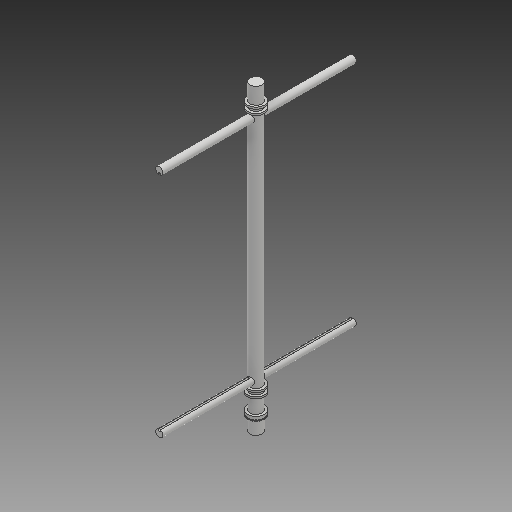
# Autodesk Inventor part: CentralBeam
Saved by Autodesk Inventor 2018 (Build 220112000, 112)
## iProperties
Created: 2016-02-23
Part Number: CentralBeam
Material: Generic
Document SubType Name: Modeling
Designer: Tore Den Store
Density: 1 g/cm^3
Appearance: Default
Author: Tore Den Store
Autodesk Inventor part; units mm, degrees
sketch "Sketch1" plane through (0, 0, 0) normal (0, 0, 1) x (1, 0, 0)
  circle A0 centre (0, 0) radius 50
  dimension "d0" = 100
  constraints: 1 centre point, 1 coincident
  measures "d0" diameter of A0
extrude "Extrusion1" add sketch "Sketch1" along normal blind 3500
ref_plane "Work Plane1" through (0, 0, 1750) normal (0, 0, -1) x (-1, 0, 0)
sketch "Sketch7" plane through (0, 0, 1750) normal (0, 0, -1) x (-1, 0, 0)
  circle A0 centre (0, 0) radius 50
  circle A1 centre (0, 0) radius 70
  constraints: 2 centre point
extrude "Extrusion6" add sketch "Sketch7" along normal blind 25
sketch "Sketch8" plane through (0, 0, 1725) normal (0, 0, -1) x (-1, 0, 0)
  circle A0 centre (0, 0) radius 70
  circle A1 centre (0, 0) radius 50
  line L0 (0, 0) -> (-2.7482, 69.946)
  line L1 (0, 0) -> (2.7482, 69.946)
  line L2 (0, 0) -> (0, 69.7958) construction
  dimension "d24" = 4.5
  dimension "d25" = 2.25
  constraints: 6 end point, 2 centre point, 2 point on circle, 1 vertical
  measures "d24" angle of L1 L0
  measures "d25" angle of L0 L2
extrude "Extrusion7" add sketch "Sketch8" along normal blind 10 contours L1 A1 L0 A0 | L1 L0 A1 picked at (0.2182, 63.3279) picked at (0, 33.3305)
ref_plane "Work Plane7" through (0, 70, 1877.5) normal (0, 1, 0) x (-1, 0, 0)
pattern_circular "Circular Pattern2" count 40 over 360 about axis through (0, 0, 0) along (0, 0, 1) of "Extrusion7"
sketch "Sketch11" plane through (0, 70, 1877.5) normal (0, 1, 0) x (-1, 0, 0)
  line L0 (0.9283, -162.5) -> (2.7482, -157.5)
  line L1 (-0.9283, -162.5) -> (-2.7482, -157.5)
  line L2 (-2.7482, -162.5) -> (2.7482, -162.5) projected
  line L3 (2.7482, -157.5) -> (2.7482, -162.5)
  line L4 (2.7482, -162.5) -> (0.9283, -162.5)
  line L5 (-2.7482, -152.5) -> (-2.7482, -162.5) projected
  line L6 (-2.7482, -157.5) -> (-2.7482, -162.5)
  line L7 (-2.7482, -162.5) -> (-0.9283, -162.5)
  point P0 (0, -1877.5)
  point P1 (2.7482, -152.5)
  dimension "d49" = 5
  dimension "d50" = 5
  dimension "d51" = 20
  dimension "d52" = 20
  constraints: 12 end point, 2 vertical, 1 collinear, 1 perpendicular
  measures "d49" distance of L5.start L1.end
  measures "d50" distance of point (2.748, -152.5) L0.end
  measures "d51" angle of L0 L3
  measures "d52" angle of L5 L1
extrude "Extrusion10" cut sketch "Sketch11" against normal up to surface round surface about axis through (0, 0, 0) along (0, 0, 1) radius 50 far side no
pattern_circular "Circular Pattern3" count 40 over 360 about axis through (0, 0, 0) along (0, 0, 1) of "Extrusion10"
ref_plane "Work Plane16" through (0, 0, 1890) normal (0, 0, 1) x (1, 0, 0)
sketch "Sketch16" plane through (0, 0, 1890) normal (0, 0, 1) x (1, 0, 0)
  circle A0 centre (0, 0) radius 50 projected
  circle A1 centre (0, 0) radius 70
  dimension "d78" = 140
  constraints: 1 centre point, 1 coincident
  measures "d78" diameter of A1
extrude "Extrusion13" add sketch "Sketch16" against normal blind 15
ref_plane "Work Plane17" through (0, 0, 1905) normal (0, 0, 1) x (1, 0, 0)
mirror "Mirror7" about plane through (0, 0, 1905) normal (0, 0, 1) of "Extrusion13"
sketch "Sketch17" plane through (0, 0, 0) normal (0, 0, -1) x (-1, 0, 0)
  circle A0 centre (0, 0) radius 50 projected
extrude "Extrusion14" cut sketch "Sketch17" against normal blind 1600
ref_plane "Work Plane18" through (0, 0, 2920) normal (0, 0, -1) x (-1, 0, 0)
mirror "Mirror8" about plane through (0, 0, 2920) normal (0, 0, -1) of "Extrusion13", "Mirror7"
sketch "Sketch18" plane through (0, 0, 3500) normal (0, 0, 1) x (1, 0, 0)
  circle A0 centre (0, 0) radius 50 projected
extrude "Extrusion15" add sketch "Sketch18" along normal blind 600
sketch "Sketch5" plane through (0, 0, 0) normal (0, 1, 0) x (-1, 0, 0)
  circle A0 centre (0, 3860) radius 30
  line L0 (50, 0) -> (50, 3500) projected
  line L1 (-70, 3905) -> (70, 3905) projected
  point P0 (0, 0)
  dimension "d12" = 60
  dimension "d13" = 50
  dimension "d88" = 45
  constraints: 1 centre point
  measures "d12" diameter of A0
  measures "d13" distance from line of L0 A0.centre
  measures "d88" distance from line of L1 A0.centre
extrude "Extrusion4" add sketch "Sketch5" along normal mid plane 1600
sketch "Sketch6" plane through (0, -800, 3860) normal (0, -1, 0) x (1, 0, 0)
  arc A0 (6.9586, -29.1818) -> (-6.9586, -29.1818) centre (0, -22) ccw
  circle A1 centre (0, 0) radius 30 projected
  arc A2 (-6.9586, -29.1818) -> (6.9586, -29.1818) centre (0, -22) ccw construction
  point P0 (0, -3860)
  dimension "d17" = 20
  dimension "d18" = 22
  constraints: 6 point on circle, 2 centre point
  measures "d17" diameter of A0
  measures "d18" distance of A0.centre A1.centre
extrude "Extrusion5" cut sketch "Sketch6" against normal up to surface contours A1 A0 round surface about axis through (0, 0, 0) along (0, 0, 1) radius 50 far side no picked at (-0.4151, -23.9651)
fillet "Fillet1" radius 0.5 2 edges at (-6.9586, -424.7567, 3830.8182) (6.9586, -424.7567, 3830.8182)
mirror "Mirror2" about plane through (0, 0, 0) normal (0, 1, 0) of "Extrusion5", "Fillet1"
mirror "Mirror9" about plane through (0, 0, 2920) normal (0, 0, -1) of "Extrusion4", "Extrusion5", "Fillet1", "Mirror2"
equation "\"d50\" = d49"
equation "\"d52\" = d51"
body "Solid1"
